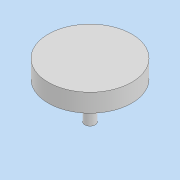
# Autodesk Inventor part: P00173-09-012
Saved by Autodesk Inventor 2022 (Build 260153070, 153G)
## iProperties
Created: 2021-07-06
Part Number: P00173-09-012
Material: Generic
Document SubType Name: Modeling
Designer: MPM
Density: 1 g/cm^3
Appearance: Default
Author: MPM
Comments: M2-Paypad 3d files for a Cardano blockchain payment terminal. Copyright (C) 2021 Maarten Menheere This program is free software; you can redistribute it and/or modify it under the terms of the GNU General Public License as published by the Free Software Foundation; either version 2 of the License, or (at your option) any later version. This program is distributed in the hope that it will be useful, but WITHOUT ANY WARRANTY; without even the implied warranty of MERCHANTABILITY or FITNESS FOR A PARTICULAR PURPOSE.  See the GNU General Public License for more details. You should have received a copy of the GNU General Public License along with this program; if not, write to the Free Software Foundation, Inc., 51 Franklin Street, Fifth Floor, Boston, MA  02110-1301, USA.
Autodesk Inventor part; units mm, degrees
ref_plane "YZ Plane" through (0, 0, 0) normal (1, 0, 0) x (0, 1, 0)
ref_plane "XZ Plane" through (0, 0, 0) normal (0, 1, 0) x (-1, 0, 0)
ref_plane "XY Plane" through (0, 0, 0) normal (0, 0, 1) x (1, 0, 0)
sketch "Sketch1" plane through (0, 0, 0) normal (0, 0, 1) x (1, 0, 0)
  line L0 (0, 0) -> (2.9, 0)
  line L1 (2.9, 0) -> (2.9, 11)
  line L2 (2.9, 11) -> (23, 20.3728)
  line L3 (0, 30.3728) -> (0, 0)
  line L4 (23, 20.3728) -> (23, 30.3728)
  line L5 (23, 30.3728) -> (0, 30.3728)
  dimension "d0" = 2.9
  dimension "d1" = 11
  dimension "d2" = 65
  dimension "d4" = 10
  dimension "d6" = 23
  constraints: 12 end point, 4 perpendicular, 1 horizontal
  measures "d0" distance of L0.start L0.end
  measures "d1" distance of L0.end L1.end
  measures "d2" angle of L1 L2
  measures "d4" distance of L2.end L4.end
  measures "d6" distance of L4.end L3.start
revolve "Revolution1" add sketch "Sketch1" angle 360 about axis through (0, 30.3728, 0) along (0, -1, 0)
body "Solid1"
